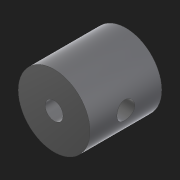
# Autodesk Inventor part: P2
Saved by Autodesk Inventor 2017 SP1 (Build 210196100, 196)
## iProperties
Created: 2018-03-20
Part Number: P2
Material: Steel
Document SubType Name: Modeling
Designer: Zach
Density: 7.85 g/cm^3
Appearance: Smooth - Black
Author: Zach
Autodesk Inventor part; units mm, degrees
ref_plane "YZ Plane" through (0, 0, 0) normal (1, 0, 0) x (0, 1, 0)
ref_plane "XZ Plane" through (0, 0, 0) normal (0, 1, 0) x (-1, 0, 0)
ref_plane "XY Plane" through (0, 0, 0) normal (0, 0, 1) x (1, 0, 0)
sketch "Sketch1" plane through (0, 0, 0) normal (0, 0, 1) x (1, 0, 0)
  circle A0 centre (0, 0) radius 4
  circle A1 centre (0, 0) radius 1
  dimension "d0" = 8
  dimension "d1" = 2
  constraints: 2 centre point, 2 coincident
  measures "d0" diameter of A0
  measures "d1" diameter of A1
extrude "Extrusion1" add sketch "Sketch1" along normal blind 8
sketch "Sketch2" plane through (0, 0, 0) normal (1, 0, 0) x (0, 1, 0)
  circle A0 centre (0, 4) radius 1
  line L0 (4, 0) -> (4, 8) projected
  line L1 (-4, 0) -> (4, 0) projected
  point P0 (0, 0)
  point P1 (4, 4)
  dimension "d4" = 2
  constraints: 1 centre point, 1 horizontal alignment, 1 midpoint, 1 vertical alignment
  measures "d4" diameter of A0
extrude "Extrusion2" cut sketch "Sketch2" along normal through all both and the other way through all
body "Solid1"
